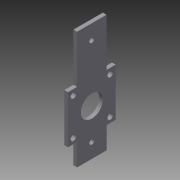
# Autodesk Inventor part: Plate
Saved by Autodesk Inventor 2014 (Build 180170000, 170)
## iProperties
Created: 2014-01-07
Part Number: Plate
Material: Generic
Document SubType Name: Modeling
Designer: Andrew Toennies
Density: 1 g/cm^3
Appearance: Default
Author: Andrew Toennies
Autodesk Inventor part; units mm, degrees
ref_plane "YZ Plane" through (0, 0, 0) normal (1, 0, 0) x (0, 1, 0)
ref_plane "XZ Plane" through (0, 0, 0) normal (0, 1, 0) x (-1, 0, 0)
ref_plane "XY Plane" through (0, 0, 0) normal (0, 0, 1) x (1, 0, 0)
sketch "Sketch1" plane through (0, 0, 0) normal (1, 0, 0) x (0, 1, 0)
  line L0 (101.6, 0) -> (101.6, -25.4)
  line L1 (0, -25.4) -> (0, 0)
  line L2 (60.2615, 7.9375) -> (18.9865, 7.9375)
  line L3 (18.9865, -33.3375) -> (60.2615, -33.3375)
  line L4 (101.6, -25.4) -> (60.2615, -25.4)
  line L5 (18.9865, 7.9375) -> (18.9865, 0)
  line L6 (18.9865, -25.4) -> (18.9865, -33.3375)
  line L7 (60.2615, 0) -> (101.6, 0)
  line L8 (60.2615, -33.3375) -> (60.2615, -25.4)
  line L9 (60.2615, 0) -> (60.2615, 7.9375)
  circle A0 centre (88.9, -12.7) radius 2.0828
  circle A1 centre (12.7, -12.7) radius 2.0828
  line L10 (55.499, 3.175) -> (23.749, 3.175) construction
  line L11 (23.749, 3.175) -> (23.749, -28.575) construction
  line L12 (23.749, -28.575) -> (55.499, -28.575) construction
  line L13 (55.499, -28.575) -> (55.499, 3.175) construction
  circle A2 centre (55.499, 3.175) radius 2.3876
  circle A3 centre (55.499, -28.575) radius 2.3876
  circle A4 centre (23.749, 3.175) radius 2.3876
  circle A5 centre (23.749, -28.575) radius 2.3876
  circle A6 centre (39.624, -12.7) radius 9.525
  line L14 (18.9865, 0) -> (0, 0)
  line L15 (0, -25.4) -> (18.9865, -25.4)
  dimension "d0" = 25.4
  dimension "d1" = 101.6
  dimension "d2" = 41.275
  dimension "d3" = 41.275
  dimension "d5" = 4.1656
  dimension "d6" = 4.1656
  dimension "d7" = 31.75
  dimension "d8" = 31.75
  dimension "d10" = 4.7625
  dimension "d11" = 12.7
  dimension "d12" = 12.7
  dimension "d13" = 12.7
  dimension "d15" = 4.7752
  dimension "d18" = 31.75
  dimension "d21" = 31.75
  dimension "d24" = 19.05
  dimension "d25" = 20.6375
  dimension "d26" = 20.6375
  dimension "d29" = 61.976
  dimension "d30" = 4.7625
  dimension "d31" = 12.7
  constraints: 32 end point, 10 parallel, 7 centre point, 5 collinear, 5 perpendicular, 4 horizontal, 1 coincident, 1 vertical, 6 other
  measures "d0" distance of L0.start L0.end
  measures "d1" distance of L0.end L1.start
  measures "d2" distance of L3.start L3.end
  measures "d3" distance between parallel lines of L3 L2
  measures "d5" diameter of A0
  measures "d6" diameter of A1
  measures "d7" distance of L12.end L10.start
  measures "d8" distance of L11.end L12.end
  measures "d10" distance between parallel lines of L9 L13
  measures "d11" distance from line of L0 A0.centre
  measures "d12" distance from line of L4 A0.centre
  measures "d13" distance from line of A1.centre L1
  measures "d15" diameter of A2
  measures "d18" distance of A2.centre A3.centre
  measures "d21" distance of A2.centre A4.centre
  measures "d24" diameter of A6
  measures "d25" distance from line of L2 A6.centre
  measures "d26" distance from line of L9 A6.centre
  measures "d29" distance from line of L0 A6.centre
  measures "d30" distance between parallel lines of L2 L10
  measures "d31" distance from line of L14 A1.centre
extrude "Extrusion1" add sketch "Sketch1" along normal blind 3.175
body "Solid1"
